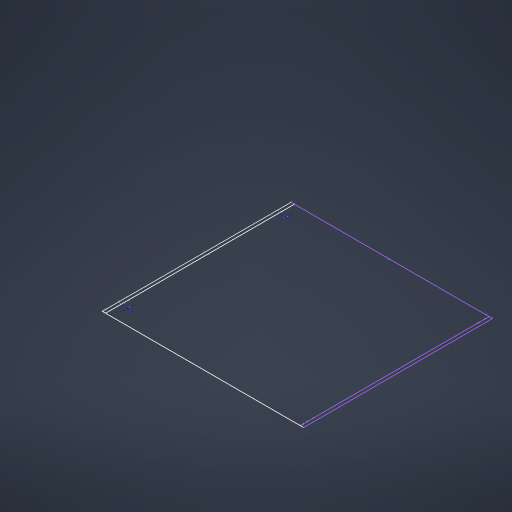
# Autodesk Inventor part: Деталь1
Saved by Autodesk Inventor 2023.4 (Build 274418000, 418)
## iProperties
Created: 2026-09-26
Part Number: Деталь1
Material: Типовые
Document SubType Name: Modeling
Designer: desig
Density: 1 g/cm^3
Appearance: По умолчанию
Author: desig
Autodesk Inventor part; units mm, degrees
ref_plane "YZ Plane" through (0, 0, 0) normal (1, 0, 0) x (0, 1, 0)
ref_plane "XZ Plane" through (0, 0, 0) normal (0, 1, 0) x (-1, 0, 0)
ref_plane "XY Plane" through (0, 0, 0) normal (0, 0, 1) x (1, 0, 0)
sketch "Эскиз1" plane through (0, 0, 0) normal (0, 1, 0) x (-1, 0, 0)
  line L0 (0, 0) -> (-16, 0)
  line L1 (-16, 0) -> (-16, -918.0582)
  line L2 (-16, -918.0582) -> (0, -918.0582)
  line L3 (0, -918.0582) -> (0, 0)
  line L4 (-962.6773, 0) -> (-978.6773, 0)
  line L5 (-978.6773, 0) -> (-978.6773, -918.0582)
  line L6 (-978.6773, -918.0582) -> (-962.6773, -918.0582)
  line L7 (-962.6773, -918.0582) -> (-962.6773, 0)
  line L8 (-16, -918.0582) -> (-962.6773, -918.0582)
  line L9 (-16, 0) -> (-962.6773, 0)
  dimension "d0" = 16
  dimension "d1" = 16
  dimension "d46" = 918.058
  dimension "d47" = 978.677
  constraints: 20 end point, 4 parallel, 3 horizontal, 3 perpendicular, 2 point on line
  measures "d0" distance of L1.end L2.end
  measures "d1" distance of L5.end L6.end
  measures "d46" distance of L2.end L0.start
  measures "d47" distance between parallel lines of L5 L3
extrude "Выдавливание1" add sketch "Эскиз1" along normal blind 500 contours L3 L2 L1 L0
extrude "Выдавливание2" add sketch "Эскиз1" against normal blind 16 from surface at 500 separate body contours L1 L8 L7 L9
extrude "Выдавливание3" add sketch "Эскиз1" along normal blind 16 separate body contours L1 L8 L7 L9
extrude "Выдавливание4" add sketch "Эскиз1" along normal up to surface (500 mm away) separate body contours L7 L6 L5 L4
sketch "DrillingSketch_1" plane through (962.6773, 484, 0) normal (1, 0, 0) x (0, 0, -1)
  line L0 (918.0582, 0) -> (0, 0) projected
  line L1 (918.0582, 0) -> (918.0582, 16) projected
  line L2 (918.0582, 16) -> (0, 16) projected
  line L3 (0, 0) -> (0, 16) projected
  line L4 (918.0582, 8) -> (0, 8) construction
  line L5 (459.0291, 8) -> (459.0291, -12) construction
  point P0 (843.0291, 8)
  point P1 (75.0291, 8)
  point P2 (811.0291, 8)
  point P3 (107.0291, 8)
  dimension "d5" = 16
  dimension "Минимальный_отступ_присадки_от_кромки_Каркас" = 70
  dimension "Long_edge_1" = 918.0582
  dimension "Расстояние_между_точками" = 768
  dimension "d733" = 32
  constraints: 5 point on line, 4 end point, 4 midpoint, 2 symmetric about line, 1 perpendicular
  measures "Long_edge_1" distance of L4.start L4.end
  measures "Расстояние_между_точками" distance of point (75.029, 8) point (843.029, 8)
  measures "d733" distance of point (843.029, 8) point (811.029, 8)
sketch "DrillingSketch_2" plane through (16, 0, -918.0582) normal (-1, 0, 0) x (0, 0, 1)
  line L0 (0, 0) -> (918.0582, 0) projected
  line L1 (918.0582, 0) -> (918.0582, 16) projected
  line L2 (0, 16) -> (918.0582, 16) projected
  line L3 (0, 0) -> (0, 16) projected
  line L4 (918.0582, 8) -> (0, 8) construction
  line L5 (459.0291, 8) -> (459.0291, -12) construction
  point P0 (843.0291, 8)
  point P1 (75.0291, 8)
  point P2 (811.0291, 8)
  point P3 (107.0291, 8)
  dimension "Минимальный_отступ_присадки_от_кромки_Каркас" = 70
  dimension "Long_edge_2" = 918.0582
  dimension "Расстояние_между_точками_2" = 768
  dimension "d736" = 32
  constraints: 5 point on line, 4 end point, 4 midpoint, 2 symmetric about line, 1 perpendicular
  measures "Long_edge_2" distance of L4.start L4.end
  measures "Расстояние_между_точками_2" distance of point (75.029, 8) point (843.029, 8)
  measures "d736" distance of point (843.029, 8) point (811.029, 8)
sketch "DrawerSketch_1" plane through (16, 484, -918.0582) normal (-1, 0, 0) x (0, 0, 1)
  line L0 (918.0582, 0) -> (0, 0) projected
  line L1 (918.0582, 16) -> (918.0582, 0) projected
  line L2 (918.0582, 16) -> (0, 16) projected
  line L3 (0, 0) -> (0, 16) projected
  line L4 (918.0582, 8) -> (0, 8) construction
  line L5 (459.0291, 8) -> (459.0291, -12) construction
  point P0 (891.0291, 8)
  point P1 (27.0291, 8)
  point P2 (859.0291, 8)
  point P3 (59.0291, 8)
  dimension "d46" = 918.058
  dimension "d47" = 978.677
  dimension "Минимальный_отступ_присадки_от_кромки_Ящик" = 20
  dimension "Long_edge_1_2" = 918.0582
  dimension "Расстояние_между_точками_3" = 864
  dimension "d739" = 32
  constraints: 5 point on line, 4 end point, 4 midpoint, 2 symmetric about line, 1 perpendicular
  measures "Long_edge_1_2" distance of L4.start L4.end
  measures "Расстояние_между_точками_3" distance of point (27.029, 8) point (891.029, 8)
  measures "d739" distance of point (891.029, 8) point (859.029, 8)
sketch "DrawerSketch_2" plane through (962.6773, 0, 0) normal (1, 0, 0) x (0, 0, -1)
  line L0 (0, 0) -> (918.0582, 0) projected
  line L1 (918.0582, 0) -> (918.0582, 16) projected
  line L2 (0, 16) -> (918.0582, 16) projected
  line L3 (0, 0) -> (0, 16) projected
  line L4 (918.0582, 8) -> (0, 8) construction
  line L5 (459.0291, 8) -> (459.0291, -12) construction
  point P0 (891.0291, 8)
  point P1 (27.0291, 8)
  point P2 (859.0291, 8)
  point P3 (59.0291, 8)
  dimension "d46" = 918.058
  dimension "d47" = 978.677
  dimension "Минимальный_отступ_присадки_от_кромки_Ящик" = 20
  dimension "Long_edge_2_2" = 918.0582
  dimension "Расстояние_между_точками_4" = 864
  dimension "d742" = 32
  constraints: 5 point on line, 4 end point, 4 midpoint, 2 symmetric about line, 1 perpendicular
  measures "Long_edge_2_2" distance of L4.start L4.end
  measures "Расстояние_между_точками_4" distance of point (27.029, 8) point (891.029, 8)
  measures "d742" distance of point (891.029, 8) point (859.029, 8)
hole "Stiajka outer 8x34" at (16, 492, -27.0291) at (16, 492, -891.0291) direction (1, 0, 0) diameter 8 depth 34 bodies 1 2 3 4
hole "Stiajka outer 5x13" at (16, 492, -27.0291) at (16, 492, -891.0291) direction (-1, 0, 0) diameter 5 depth 13 bodies 1 2 3 4
hole "Stiajka inner 8x10" at (16, 492, -59.0291) at (16, 492, -859.0291) direction (-1, 0, 0) diameter 8 depth 10 bodies 1 2 3 4
hole "Stiajka inner 8x20" at (16, 492, -59.0291) at (16, 492, -859.0291) direction (1, 0, 0) diameter 8 depth 20 bodies 1 2 3 4
sketch "StiajkaSideSketch" plane through (16, 484, 0) normal (0, -1, 0) x (1, 0, 0)
  line L0 (0, -31.0291) -> (0, -23.0291) projected
  line L1 (34, -23.0291) -> (34, -31.0291) projected
  line L2 (0, -895.0291) -> (0, -887.0291) projected
  line L3 (34, -887.0291) -> (34, -895.0291) projected
  point P0 (34, -27.0291)
  point P1 (34, -891.0291)
  dimension "d46" = 918.058
  dimension "d47" = 978.677
  constraints: 2 midpoint
hole "Stiajka cup" at (50, 484, -27.0291) at (50, 484, -891.0291) direction (0, 1, 0) diameter 15 depth 12.5 bodies 1 2 3 4
hole "Stiajka outer 8x34 2" at (962.6773, 8, -891.0291) at (962.6773, 8, -27.0291) direction (-1, 0, 0) diameter 8 depth 34 bodies 1 2 3 4
hole "Stiajka outer 5x13 2" at (962.6773, 8, -891.0291) at (962.6773, 8, -27.0291) direction (1, 0, 0) diameter 5 depth 13 bodies 1 2 3 4
hole "Stiajka inner 8x10 2" at (962.6773, 8, -859.0291) at (962.6773, 8, -59.0291) direction (1, 0, 0) diameter 8 depth 10 bodies 1 2 3 4
hole "Stiajka inner 8x20 2" at (962.6773, 8, -859.0291) at (962.6773, 8, -59.0291) direction (-1, 0, 0) diameter 8 depth 20 bodies 1 2 3 4
sketch "StiajkaSideSketch_2" plane through (0, 0, 0) normal (0, -1, 0) x (1, 0, 0)
  line L0 (962.6773, -887.0291) -> (962.6773, -895.0291) projected
  line L1 (928.6773, -895.0291) -> (928.6773, -887.0291) projected
  line L2 (962.6773, -23.0291) -> (962.6773, -31.0291) projected
  line L3 (928.6773, -31.0291) -> (928.6773, -23.0291) projected
  point P0 (928.6773, -891.0291)
  point P1 (928.6773, -27.0291)
  dimension "d46" = 918.058
  dimension "d47" = 978.677
  constraints: 2 midpoint
hole "Stiajka cup 2" at (928.6773, 0, -891.0291) at (928.6773, 0, -27.0291) direction (0, 1, 0) diameter 15 depth 12.5 bodies 1 2 3 4
hole "Confirmat 5mm inward" at (962.6773, 492, -843.0291) at (962.6773, 492, -459.0291) at (962.6773, 492, -75.0291) direction (1, 0, 0) diameter 5 depth 20 bodies 1 2 3 4
hole "Confirmat 3mm outward" at (962.6773, 492, -843.0291) at (962.6773, 492, -459.0291) at (962.6773, 492, -75.0291) direction (-1, 0, 0) diameter 3 depth 50 bodies 1 2 3 4
hole "Stiajka outer 8x34 3" at (16, 8, -75.0291) at (16, 8, -843.0291) direction (1, 0, 0) diameter 8 depth 34 bodies 1 2 3 4
hole "Stiajka outer 5x13 3" at (16, 8, -75.0291) at (16, 8, -843.0291) direction (-1, 0, 0) diameter 5 depth 13 bodies 1 2 3 4
hole "Stiajka inner 8x10 3" at (16, 8, -107.0291) at (16, 8, -811.0291) direction (-1, 0, 0) diameter 8 depth 10 bodies 1 2 3 4
hole "Stiajka inner 8x20 3" at (16, 8, -107.0291) at (16, 8, -811.0291) direction (1, 0, 0) diameter 8 depth 20 bodies 1 2 3 4
sketch "StiajkaSideSketch_3" plane through (0, 0, 0) normal (0, -1, 0) x (1, 0, 0)
  line L0 (16, -79.0291) -> (16, -71.0291) projected
  line L1 (50, -71.0291) -> (50, -79.0291) projected
  line L2 (16, -847.0291) -> (16, -839.0291) projected
  line L3 (50, -839.0291) -> (50, -847.0291) projected
  point P0 (50, -75.0291)
  point P1 (50, -843.0291)
  dimension "d46" = 918.058
  dimension "d47" = 978.677
  constraints: 2 midpoint
hole "Stiajka cup 3" [suppressed]
sketch "Эскиз56" plane through (0, 16, 0) normal (0, 1, 0) x (1, 0, 0)
  point P0 (0, 0)
  point P1 (50, 71.0291)
  point P2 (50, 839.0291)
  dimension "d46" = 918.058
  dimension "d47" = 978.677
hole "Отверстие102" at (50, 16, -839.0291) at (50, 16, -71.0291) direction (0, -1, 0) diameter 15 depth 13 bodies 3
equation "\"d0\" = Толщина_каркаса"
equation "\"d1\" = Толщина_каркаса"
equation "\"d5\" = Толщина_каркаса"
equation "\"d7\" = Толщина_каркаса"
equation "\"Минимальный_отступ_присадки_от_кромки_Каркас\" = 70"
equation "\"Минимальный_отступ_присадки_от_кромки_Ящик\" = 20"
equation "\"d771\" = Стяжка_D"
equation "\"d776\" = Стяжка_h"
equation "\"d806\" = Стяжка_D"
equation "\"d811\" = Стяжка_h"
equation "\"d855\" = Стяжка_D"
equation "\"d860\" = Стяжка_h"
equation "\"d862\" = Стяжка_D"
equation "\"Толщина_каркаса\" = 16"
equation "\"Стяжка_D\" = 15"
equation "\"Стяжка_h\" = 12.5"
equation "\"Стяжка_D_резьбыШтока\" = 5"
equation "\"Стяжка_D_телаШтока\" = 8"
equation "\"Стяжка_резьбыШтока_Петля_h\" = 12.5"
equation "\"Стяжка_отступ\" = 34"
equation "\"Конфирмат_D_вПласть\" = 8"
equation "\"Конфирмат_D_вТорец\" = 5"
equation "\"Толщина_каркаса_ящика\" = 16"
equation "\"Шкант_D\" = 8"
equation "\"Полкодержатель_D\" = 5"
equation "\"Полкодержатель_смещение_от_низа_полки\" = 5"
equation "\"Петля_D_присадки\" = 35"
equation "\"M_Конфирмат_глубина_резьбы\" = 35"
equation "\"M_Конфирмат_D_вПласть\" = 5"
equation "\"M_Конфирмат_D_вТорец\" = 3"
equation "\"Толщина_задн_ст_Володя\" = 3"
equation "\"Толщина_дна_ящика_Володя\" = 6"
equation "\"Минимальное_расстояния_от_заднСт_ящика_до_заднСт\" = 25"
equation "\"Западание_кромки_полки_за_каркас\" = 5"
